Autodesk Fusion 360 part; units mm, degrees
note: some values were not read from the file. Set by a fixed rule: which sketch regions a step uses.
(part 12 of 20)
  spline S66 degree 5 poles (-5.1346, 28.5878) (-5.1347, 28.5879) (-5.1347, 28.5881) (-5.1348, 28.5884) (-5.1349, 28.5889) (-5.135, 28.5896) (-5.1352, 28.5905) (-5.1354, 28.5915) (-5.1356, 28.5925) (-5.1358, 28.5937) (-5.1361, 28.595) (-5.1363, 28.5964) (-5.1367, 28.5979) (-5.137, 28.5995) (-5.1374, 28.6012) (-5.1377, 28.603) (-5.1381, 28.6049) (-5.1386, 28.6069) (-5.139, 28.6089) (-5.1395, 28.6111) (-5.14, 28.6134) (-5.1406, 28.6158) (-5.1411, 28.6182) (-5.1417, 28.6208) (-5.1423, 28.6234) (-5.143, 28.6262) (-5.1436, 28.629) (-5.1443, 28.6319) (-5.145, 28.6349) (-5.1458, 28.6379) (-5.1465, 28.6411) (-5.1473, 28.6443) (-5.1481, 28.6477) (-5.149, 28.6511) (-5.1499, 28.6545) (-5.1508, 28.6581) (-5.1517, 28.6617) (-5.1527, 28.6655) (-5.1536, 28.6693) (-5.1546, 28.6731) (-5.1557, 28.6771) (-5.1567, 28.6811) (-5.1578, 28.6852) (-5.1589, 28.6893) (-5.1601, 28.6936) (-5.1613, 28.6979) (-5.1625, 28.7023) (-5.1637, 28.7067) (-5.1649, 28.7112) (-5.1662, 28.7158) (-5.1675, 28.7205) (-5.1689, 28.7252) (-5.1702, 28.73) (-5.1716, 28.7349) (-5.173, 28.7398) (-5.1745, 28.7448) (-5.176, 28.7498) (-5.1775, 28.7549) (-5.179, 28.7601) (-5.1806, 28.7654) (-5.1822, 28.7707) (-5.1838, 28.776) (-5.1854, 28.7815) (-5.1871, 28.7869) (-5.1888, 28.7925) (-5.1905, 28.7981) (-5.1923, 28.8038) (-5.1941, 28.8095) (-5.1959, 28.8153) (-5.1978, 28.8211) (-5.1996, 28.827) (-5.2015, 28.833) (-5.2035, 28.839) (-5.2054, 28.8451) (-5.2074, 28.8512) (-5.2094, 28.8573) (-5.2115, 28.8636) (-5.2136, 28.8699) (-5.2157, 28.8762) (-5.2178, 28.8826) (-5.22, 28.889) (-5.2222, 28.8955) (-5.2244, 28.9021) (-5.2266, 28.9087) (-5.2289, 28.9153) (-5.2312, 28.922) (-5.2336, 28.9288) (-5.2359, 28.9356) (-5.2383, 28.9424) (-5.2408, 28.9493) (-5.2432, 28.9563) (-5.2457, 28.9633) (-5.2482, 28.9703) (-5.2508, 28.9774) (-5.2533, 28.9846) (-5.2559, 28.9918) (-5.2586, 28.999) (-5.2612, 29.0063) (-5.2639, 29.0136) (-5.2666, 29.021) (-5.2694, 29.0284) (-5.2722, 29.0358) (-5.275, 29.0433) (-5.2778, 29.0509) (-5.2807, 29.0585) (-5.2836, 29.0661) (-5.2865, 29.0738) (-5.2895, 29.0815) (-5.2925, 29.0893) (-5.2955, 29.0971) (-5.2986, 29.105) (-5.3016, 29.1129) (-5.3047, 29.1208) (-5.3079, 29.1288) (-5.3111, 29.1368) (-5.3143, 29.1448) (-5.3175, 29.1529) (-5.3207, 29.1611) (-5.324, 29.1692) (-5.3273, 29.1775) (-5.3307, 29.1857) (-5.3341, 29.194) (-5.3375, 29.2023) (-5.3409, 29.2107) (-5.3444, 29.2191) (-5.3479, 29.2276) (-5.3514, 29.2361) (-5.355, 29.2446) (-5.3586, 29.2531) (-5.3622, 29.2617) (-5.3658, 29.2704) (-5.3695, 29.279) (-5.3732, 29.2878) (-5.377, 29.2965) (-5.3807, 29.3053) (-5.3846, 29.3141) (-5.3884, 29.3229) (-5.3922, 29.3318) (-5.3961, 29.3407) (-5.4001, 29.3497) (-5.404, 29.3587) (-5.408, 29.3677) (-5.412, 29.3767) (-5.4161, 29.3858) (-5.4201, 29.395) (-5.4242, 29.4041) (-5.4284, 29.4133) (-5.4325, 29.4225) (-5.4367, 29.4318) (-5.441, 29.441) (-5.4452, 29.4504) (-5.4495, 29.4597) (-5.4538, 29.4691) (-5.4582, 29.4785) (-5.4625, 29.4879) (-5.467, 29.4974) (-5.4714, 29.5069) (-5.4759, 29.5165) (-5.4804, 29.526) (-5.4849, 29.5356) (-5.4895, 29.5452) (-5.494, 29.5549) (-5.4987, 29.5646) (-5.5033, 29.5743) (-5.508, 29.584) (-5.5127, 29.5938) (-5.5175, 29.6036) (-5.5222, 29.6134) (-5.527, 29.6233) (-5.5319, 29.6332) (-5.5367, 29.6431) (-5.5416, 29.653) (-5.5466, 29.663) (-5.5515, 29.673) (-5.5565, 29.683) (-5.5615, 29.6931) (-5.5666, 29.7032) (-5.5717, 29.7133) (-5.5768, 29.7234) (-5.5819, 29.7336) (-5.5871, 29.7437) (-5.5923, 29.754) (-5.5975, 29.7642) (-5.6028, 29.7745) (-5.6081, 29.7847) (-5.6134, 29.7951) (-5.6188, 29.8054) (-5.6242, 29.8158) (-5.6296, 29.8262) (-5.635, 29.8366) (-5.6405, 29.847) (-5.646, 29.8575) (-5.6515, 29.868) (-5.6571, 29.8785) (-5.6627, 29.889) (-5.6683, 29.8996) (-5.674, 29.9102) (-5.6797, 29.9208) (-5.6854, 29.9314) (-5.6912, 29.9421) (-5.697, 29.9527) (-5.7028, 29.9634) (-5.7086, 29.9742) (-5.7145, 29.9849) (-5.7204, 29.9957) (-5.7263, 30.0065) (-5.7323, 30.0173) (-5.7383, 30.0281) (-5.7443, 30.039) (-5.7504, 30.0499) (-5.7565, 30.0608) (-5.7626, 30.0717) (-5.7688, 30.0826) (-5.7749, 30.0936) (-5.7811, 30.1046) (-5.7874, 30.1156) (-5.7937, 30.1266) (-5.8, 30.1377) (-5.8063, 30.1487) (-5.8127, 30.1598) (-5.8191, 30.1709) (-5.8255, 30.1821) (-5.8319, 30.1932) (-5.8384, 30.2044) (-5.8449, 30.2156) (-5.8515, 30.2268) (-5.8581, 30.238) (-5.8647, 30.2492) (-5.8713, 30.2605) (-5.878, 30.2718) (-5.8847, 30.2831) (-5.8914, 30.2944) (-5.8982, 30.3058) (-5.905, 30.3171) (-5.9118, 30.3285) (-5.9187, 30.3399) (-5.9255, 30.3513) (-5.9325, 30.3628) (-5.9394, 30.3742) (-5.9464, 30.3857) (-5.9534, 30.3972) (-5.959, 30.4064) (-5.9633, 30.4133) (-5.9661, 30.4179) (-5.9675, 30.4202) knots 0 0 0 0 0 0 0.00416667 0.00833333 0.0125 0.01666667 0.02083333 0.025 0.02916667 0.03333333 0.0375 0.04166667 0.04583333 0.05 0.05416667 0.05833333 0.0625 0.06666667 0.07083333 0.075 0.07916667 0.08333333 0.0875 0.09166667 0.09583333 0.1 0.10416667 0.10833333 0.1125 0.11666667 0.12083333 0.125 0.12916667 0.13333333 0.1375 0.14166667 0.14583333 0.15 0.15416667 0.15833333 0.1625 0.16666667 0.17083333 0.175 0.17916667 0.18333333 0.1875 0.19166667 0.19583333 0.2 0.20416667 0.20833333 0.2125 0.21666667 0.22083333 0.225 0.22916667 0.23333333 0.2375 0.24166667 0.24583333 0.25 0.25416667 0.25833333 0.2625 0.26666667 0.27083333 0.275 0.27916667 0.28333333 0.2875 0.29166667 0.29583333 0.3 0.30416667 0.30833333 0.3125 0.31666667 0.32083333 0.325 0.32916667 0.33333333 0.3375 0.34166667 0.34583333 0.35 0.35416667 0.35833333 0.3625 0.36666667 0.37083333 0.375 0.37916667 0.38333333 0.3875 0.39166667 0.39583333 0.4 0.40416667 0.40833333 0.4125 0.41666667 0.42083333 0.425 0.42916667 0.43333333 0.4375 0.44166667 0.44583333 0.45 0.45416667 0.45833333 0.4625 0.46666667 0.47083333 0.475 0.47916667 0.48333333 0.4875 0.49166667 0.49583333 0.5 0.50416667 0.50833333 0.5125 0.51666667 0.52083333 0.525 0.52916667 0.53333333 0.5375 0.54166667 0.54583333 0.55 0.55416667 0.55833333 0.5625 0.56666667 0.57083333 0.575 0.57916667 0.58333333 0.5875 0.59166667 0.59583333 0.6 0.60416667 0.60833333 0.6125 0.61666667 0.62083333 0.625 0.62916667 0.63333333 0.6375 0.64166667 0.64583333 0.65 0.65416667 0.65833333 0.6625 0.66666667 0.67083333 0.675 0.67916667 0.68333333 0.6875 0.69166667 0.69583333 0.7 0.70416667 0.70833333 0.7125 0.71666667 0.72083333 0.725 0.72916667 0.73333333 0.7375 0.74166667 0.74583333 0.75 0.75416667 0.75833333 0.7625 0.76666667 0.77083333 0.775 0.77916667 0.78333333 0.7875 0.79166667 0.79583333 0.8 0.80416667 0.80833333 0.8125 0.81666667 0.82083333 0.825 0.82916667 0.83333333 0.8375 0.84166667 0.84583333 0.85 0.85416667 0.85833333 0.8625 0.86666667 0.87083333 0.875 0.87916667 0.88333333 0.8875 0.89166667 0.89583333 0.9 0.90416667 0.90833333 0.9125 0.91666667 0.92083333 0.925 0.92916667 0.93333333 0.9375 0.94166667 0.94583333 0.95 0.95416667 0.95833333 0.9625 0.96666667 0.97083333 0.975 0.97916667 0.98333333 0.9875 0.99166667 0.99583333 1 1 1 1 1 1
  spline S67 degree 5 poles (-15.9204, 26.5997) (-15.9199, 26.597) (-15.9189, 26.5917) (-15.9174, 26.5837) (-15.9154, 26.5731) (-15.913, 26.5599) (-15.9105, 26.5467) (-15.908, 26.5335) (-15.9055, 26.5204) (-15.9029, 26.5073) (-15.9004, 26.4943) (-15.8979, 26.4812) (-15.8953, 26.4682) (-15.8927, 26.4553) (-15.8902, 26.4424) (-15.8876, 26.4295) (-15.885, 26.4166) (-15.8824, 26.4038) (-15.8798, 26.391) (-15.8771, 26.3783) (-15.8745, 26.3656) (-15.8719, 26.3529) (-15.8692, 26.3403) (-15.8666, 26.3276) (-15.8639, 26.3151) (-15.8612, 26.3025) (-15.8585, 26.29) (-15.8558, 26.2776) (-15.8531, 26.2651) (-15.8504, 26.2528) (-15.8477, 26.2404) (-15.8449, 26.2281) (-15.8422, 26.2158) (-15.8394, 26.2035) (-15.8367, 26.1913) (-15.8339, 26.1792) (-15.8311, 26.167) (-15.8283, 26.1549) (-15.8255, 26.1428) (-15.8227, 26.1308) (-15.8199, 26.1188) (-15.8171, 26.1069) (-15.8143, 26.095) (-15.8115, 26.0831) (-15.8086, 26.0712) (-15.8058, 26.0594) (-15.8029, 26.0477) (-15.8001, 26.0359) (-15.7972, 26.0242) (-15.7943, 26.0126) (-15.7914, 26.001) (-15.7886, 25.9894) (-15.7857, 25.9778) (-15.7828, 25.9663) (-15.7798, 25.9549) (-15.7769, 25.9435) (-15.774, 25.9321) (-15.7711, 25.9207) (-15.7682, 25.9094) (-15.7652, 25.8982) (-15.7623, 25.8869) (-15.7593, 25.8757) (-15.7564, 25.8646) (-15.7534, 25.8535) (-15.7504, 25.8424) (-15.7475, 25.8314) (-15.7445, 25.8204) (-15.7415, 25.8094) (-15.7385, 25.7985) (-15.7355, 25.7877) (-15.7325, 25.7768) (-15.7295, 25.766) (-15.7265, 25.7553) (-15.7235, 25.7446) (-15.7205, 25.7339) (-15.7175, 25.7233) (-15.7145, 25.7127) (-15.7114, 25.7022) (-15.7084, 25.6917) (-15.7054, 25.6812) (-15.7023, 25.6708) (-15.6993, 25.6604) (-15.6963, 25.6501) (-15.6932, 25.6398) (-15.6902, 25.6296) (-15.6871, 25.6194) (-15.6841, 25.6092) (-15.681, 25.5991) (-15.6779, 25.589) (-15.6749, 25.579) (-15.6718, 25.569) (-15.6688, 25.559) (-15.6657, 25.5491) (-15.6626, 25.5393) (-15.6596, 25.5294) (-15.6565, 25.5197) (-15.6534, 25.5099) (-15.6503, 25.5003) (-15.6473, 25.4906) (-15.6442, 25.481) (-15.6411, 25.4715) (-15.638, 25.462) (-15.635, 25.4525) (-15.6319, 25.4431) (-15.6288, 25.4337) (-15.6257, 25.4244) (-15.6227, 25.4151) (-15.6196, 25.4059) (-15.6165, 25.3967) (-15.6134, 25.3876) (-15.6104, 25.3785) (-15.6073, 25.3694) (-15.6042, 25.3604) (-15.6012, 25.3515) (-15.5981, 25.3426) (-15.595, 25.3337) (-15.592, 25.3249) (-15.5889, 25.3161) (-15.5859, 25.3074) (-15.5828, 25.2988) (-15.5798, 25.2901) (-15.5767, 25.2816) (-15.5737, 25.2731) (-15.5706, 25.2646) (-15.5676, 25.2562) (-15.5645, 25.2478) (-15.5615, 25.2394) (-15.5585, 25.2312) (-15.5555, 25.2229) (-15.5524, 25.2148) (-15.5494, 25.2066) (-15.5464, 25.1986) (-15.5434, 25.1905) (-15.5404, 25.1826) (-15.5374, 25.1746) (-15.5344, 25.1668) (-15.5315, 25.1589) (-15.5285, 25.1512) (-15.5255, 25.1434) (-15.5226, 25.1358) (-15.5196, 25.1282) (-15.5166, 25.1206) (-15.5137, 25.1131) (-15.5108, 25.1056) (-15.5078, 25.0982) (-15.5049, 25.0909) (-15.502, 25.0836) (-15.4991, 25.0763) (-15.4962, 25.0691) (-15.4933, 25.062) (-15.4905, 25.0549) (-15.4876, 25.0479) (-15.4848, 25.0409) (-15.4819, 25.034) (-15.4791, 25.0271) (-15.4762, 25.0203) (-15.4734, 25.0136) (-15.4706, 25.0069) (-15.4678, 25.0002) (-15.4651, 24.9936) (-15.4623, 24.9871) (-15.4595, 24.9806) (-15.4568, 24.9742) (-15.4541, 24.9679) (-15.4514, 24.9616) (-15.4486, 24.9553) (-15.446, 24.9492) (-15.4433, 24.943) (-15.4406, 24.937) (-15.438, 24.931) (-15.4353, 24.925) (-15.4327, 24.9192) (-15.4301, 24.9133) (-15.4275, 24.9076) (-15.425, 24.9019) (-15.4224, 24.8962) (-15.4199, 24.8907) (-15.4174, 24.8852) (-15.4149, 24.8797) (-15.4124, 24.8743) (-15.4099, 24.869) (-15.4075, 24.8637) (-15.405, 24.8585) (-15.4026, 24.8534) (-15.4002, 24.8483) (-15.3979, 24.8433) (-15.3955, 24.8384) (-15.3932, 24.8335) (-15.3909, 24.8287) (-15.3886, 24.8239) (-15.3863, 24.8193) (-15.3841, 24.8147) (-15.3819, 24.8101) (-15.3797, 24.8056) (-15.3775, 24.8012) (-15.3754, 24.7969) (-15.3733, 24.7926) (-15.3712, 24.7884) (-15.3691, 24.7843) (-15.3671, 24.7802) (-15.3651, 24.7763) (-15.3631, 24.7723) (-15.3611, 24.7685) (-15.3592, 24.7647) (-15.3573, 24.761) (-15.3554, 24.7574) (-15.3536, 24.7539) (-15.3518, 24.7504) (-15.35, 24.747) (-15.3482, 24.7437) (-15.3465, 24.7404) (-15.3449, 24.7372) (-15.3432, 24.7341) (-15.3416, 24.7311) (-15.34, 24.7282) (-15.3385, 24.7253) (-15.337, 24.7225) (-15.3355, 24.7198) (-15.3341, 24.7172) (-15.3327, 24.7147) (-15.3313, 24.7122) (-15.33, 24.7099) (-15.3287, 24.7076) (-15.3275, 24.7054) (-15.3263, 24.7033) (-15.3252, 24.7012) (-15.3241, 24.6993) (-15.323, 24.6974) (-15.322, 24.6956) (-15.321, 24.694) (-15.3201, 24.6924) (-15.3193, 24.6909) (-15.3184, 24.6895) (-15.3177, 24.6881) (-15.3169, 24.6869) (-15.3163, 24.6858) (-15.3157, 24.6848) (-15.3151, 24.6838) (-15.3146, 24.683) (-15.3142, 24.6822) (-15.3138, 24.6816) (-15.3135, 24.6812) (-15.3133, 24.6809) (-15.3132, 24.6807) (-15.3132, 24.6806) knots -1 -1 -1 -1 -1 -1 -0.99583333 -0.99166667 -0.9875 -0.98333333 -0.97916667 -0.975 -0.97083333 -0.96666667 -0.9625 -0.95833333 -0.95416667 -0.95 -0.94583333 -0.94166667 -0.9375 -0.93333333 -0.92916667 -0.925 -0.92083333 -0.91666667 -0.9125 -0.90833333 -0.90416667 -0.9 -0.89583333 -0.89166667 -0.8875 -0.88333333 -0.87916667 -0.875 -0.87083333 -0.86666667 -0.8625 -0.85833333 -0.85416667 -0.85 -0.84583333 -0.84166667 -0.8375 -0.83333333 -0.82916667 -0.825 -0.82083333 -0.81666667 -0.8125 -0.80833333 -0.80416667 -0.8 -0.79583333 -0.79166667 -0.7875 -0.78333333 -0.77916667 -0.775 -0.77083333 -0.76666667 -0.7625 -0.75833333 -0.75416667 -0.75 -0.74583333 -0.74166667 -0.7375 -0.73333333 -0.72916667 -0.725 -0.72083333 -0.71666667 -0.7125 -0.70833333 -0.70416667 -0.7 -0.69583333 -0.69166667 -0.6875 -0.68333333 -0.67916667 -0.675 -0.67083333 -0.66666667 -0.6625 -0.65833333 -0.65416667 -0.65 -0.64583333 -0.64166667 -0.6375 -0.63333333 -0.62916667 -0.625 -0.62083333 -0.61666667 -0.6125 -0.60833333 -0.60416667 -0.6 -0.59583333 -0.59166667 -0.5875 -0.58333333 -0.57916667 -0.575 -0.57083333 -0.56666667 -0.5625 -0.55833333 -0.55416667 -0.55 -0.54583333 -0.54166667 -0.5375 -0.53333333 -0.52916667 -0.525 -0.52083333 -0.51666667 -0.5125 -0.50833333 -0.50416667 -0.5 -0.49583333 -0.49166667 -0.4875 -0.48333333 -0.47916667 -0.475 -0.47083333 -0.46666667 -0.4625 -0.45833333 -0.45416667 -0.45 -0.44583333 -0.44166667 -0.4375 -0.43333333 -0.42916667 -0.425 -0.42083333 -0.41666667 -0.4125 -0.40833333 -0.40416667 -0.4 -0.39583333 -0.39166667 -0.3875 -0.38333333 -0.37916667 -0.375 -0.37083333 -0.36666667 -0.3625 -0.35833333 -0.35416667 -0.35 -0.34583333 -0.34166667 -0.3375 -0.33333333 -0.32916667 -0.325 -0.32083333 -0.31666667 -0.3125 -0.30833333 -0.30416667 -0.3 -0.29583333 -0.29166667 -0.2875 -0.28333333 -0.27916667 -0.275 -0.27083333 -0.26666667 -0.2625 -0.25833333 -0.25416667 -0.25 -0.24583333 -0.24166667 -0.2375 -0.23333333 -0.22916667 -0.225 -0.22083333 -0.21666667 -0.2125 -0.20833333 -0.20416667 -0.2 -0.19583333 -0.19166667 -0.1875 -0.18333333 -0.17916667 -0.175 -0.17083333 -0.16666667 -0.1625 -0.15833333 -0.15416667 -0.15 -0.14583333 -0.14166667 -0.1375 -0.13333333 -0.12916667 -0.125 -0.12083333 -0.11666667 -0.1125 -0.10833333 -0.10416667 -0.1 -0.09583333 -0.09166667 -0.0875 -0.08333333 -0.07916667 -0.075 -0.07083333 -0.06666667 -0.0625 -0.05833333 -0.05416667 -0.05 -0.04583333 -0.04166667 -0.0375 -0.03333333 -0.02916667 -0.025 -0.02083333 -0.01666667 -0.0125 -0.00833333 -0.00416667 0 0 0 0 0 0
  line L145 (-2.1183, -28.9679) -> (-2.1182, -28.9671)
  line L146 (-3.9507, -28.7745) -> (-3.9508, -28.7753)
  line L147 (25.6012, 13.7171) -> (25.6019, 13.7175)
  line L148 (26.1461, 12.6495) -> (26.1453, 12.6491)
  arc A66 (-5.0824, -28.2972) -> (-3.9106, -28.4828) centre (0, 0) ccw
  arc A67 (-3.7249, -30.7754) -> (-2.755, -30.8773) centre (0, 0) ccw
  spline S68 degree 5 poles (-16.3184, 24.0278) (-16.3185, 24.0279) (-16.3186, 24.0281) (-16.3188, 24.0283) (-16.3191, 24.0287) (-16.3195, 24.0294) (-16.32, 24.0301) (-16.3206, 24.0309) (-16.3212, 24.0317) (-16.3219, 24.0327) (-16.3227, 24.0338) (-16.3235, 24.035) (-16.3244, 24.0362) (-16.3253, 24.0375) (-16.3263, 24.0389) (-16.3274, 24.0404) (-16.3286, 24.042) (-16.3298, 24.0436) (-16.331, 24.0453) (-16.3324, 24.0471) (-16.3338, 24.049) (-16.3352, 24.051) (-16.3367, 24.053) (-16.3383, 24.0551) (-16.3399, 24.0572) (-16.3416, 24.0595) (-16.3434, 24.0618) (-16.3452, 24.0641) (-16.3471, 24.0666) (-16.349, 24.0691) (-16.351, 24.0717) (-16.353, 24.0743) (-16.3551, 24.077) (-16.3573, 24.0798) (-16.3595, 24.0826) (-16.3618, 24.0855) (-16.3641, 24.0884) (-16.3665, 24.0914) (-16.3689, 24.0945) (-16.3714, 24.0976) (-16.374, 24.1008) (-16.3766, 24.104) (-16.3792, 24.1073) (-16.3819, 24.1107) (-16.3847, 24.1141) (-16.3875, 24.1176) (-16.3904, 24.1211) (-16.3933, 24.1246) (-16.3963, 24.1283) (-16.3994, 24.1319) (-16.4024, 24.1356) (-16.4056, 24.1394) (-16.4088, 24.1432) (-16.412, 24.1471) (-16.4153, 24.151) (-16.4187, 24.155) (-16.4221, 24.159) (-16.4256, 24.1631) (-16.4291, 24.1672) (-16.4326, 24.1713) (-16.4362, 24.1755) (-16.4399, 24.1798) (-16.4436, 24.1841) (-16.4474, 24.1884) (-16.4512, 24.1928) (-16.455, 24.1972) (-16.459, 24.2017) (-16.4629, 24.2062) (-16.4669, 24.2107) (-16.471, 24.2153) (-16.4751, 24.2199) (-16.4793, 24.2246) (-16.4835, 24.2293) (-16.4877, 24.234) (-16.492, 24.2388) (-16.4964, 24.2436) (-16.5008, 24.2485) (-16.5053, 24.2534) (-16.5098, 24.2583) (-16.5143, 24.2633) (-16.5189, 24.2683) (-16.5236, 24.2733) (-16.5282, 24.2784) (-16.533, 24.2835) (-16.5378, 24.2887) (-16.5426, 24.2939) (-16.5475, 24.2991) (-16.5524, 24.3043) (-16.5574, 24.3096) (-16.5624, 24.3149) (-16.5675, 24.3203) (-16.5726, 24.3257) (-16.5778, 24.3311) (-16.583, 24.3365) (-16.5882, 24.342) (-16.5935, 24.3475) (-16.5989, 24.353) (-16.6043, 24.3586) (-16.6097, 24.3642) (-16.6152, 24.3698) (-16.6207, 24.3755) (-16.6263, 24.3812) (-16.6319, 24.3869) (-16.6376, 24.3926) (-16.6433, 24.3984) (-16.6491, 24.4042) (-16.6549, 24.41) (-16.6607, 24.4159) (-16.6666, 24.4218) (-16.6725, 24.4277) (-16.6785, 24.4336) (-16.6845, 24.4395) (-16.6906, 24.4455) (-16.6967, 24.4515) (-16.7029, 24.4576) (-16.7091, 24.4636) (-16.7153, 24.4697) (-16.7216, 24.4758) (-16.7279, 24.482) (-16.7343, 24.4881) (-16.7407, 24.4943) (-16.7472, 24.5005) (-16.7537, 24.5067) (-16.7602, 24.513) (-16.7668, 24.5192) (-16.7735, 24.5255) (-16.7801, 24.5319) (-16.7869, 24.5382) (-16.7936, 24.5446) (-16.8004, 24.5509) (-16.8073, 24.5573) (-16.8142, 24.5638) (-16.8211, 24.5702) (-16.8281, 24.5767) (-16.8351, 24.5831) (-16.8421, 24.5897) (-16.8492, 24.5962) (-16.8564, 24.6027) (-16.8636, 24.6093) (-16.8708, 24.6159) (-16.8781, 24.6225) (-16.8854, 24.6291) (-16.8927, 24.6357) (-16.9001, 24.6424) (-16.9075, 24.6491) (-16.915, 24.6558) (-16.9225, 24.6625) (-16.9301, 24.6692) (-16.9377, 24.6759) (-16.9453, 24.6827) (-16.953, 24.6895) (-16.9607, 24.6963) (-16.9685, 24.7031) (-16.9763, 24.7099) (-16.9841, 24.7168) (-16.992, 24.7236) (-16.9999, 24.7305) (-17.0079, 24.7374) (-17.0159, 24.7443) (-17.0239, 24.7512) (-17.032, 24.7582) (-17.0401, 24.7651) (-17.0483, 24.7721) (-17.0565, 24.7791) (-17.0647, 24.7861) (-17.073, 24.7931) (-17.0813, 24.8001) (-17.0897, 24.8071) (-17.0981, 24.8142) (-17.1065, 24.8212) (-17.115, 24.8283) (-17.1235, 24.8354) (-17.1321, 24.8425) (-17.1407, 24.8496) (-17.1493, 24.8568) (-17.158, 24.8639) (-17.1667, 24.8711) (-17.1754, 24.8782) (-17.1842, 24.8854) (-17.1931, 24.8926) (-17.2019, 24.8998) (-17.2108, 24.907) (-17.2198, 24.9142) (-17.2288, 24.9215) (-17.2378, 24.9287) (-17.2469, 24.936) (-17.2559, 24.9432) (-17.2651, 24.9505) (-17.2743, 24.9578) (-17.2835, 24.9651) (-17.2927, 24.9724) (-17.302, 24.9797) (-17.3113, 24.9871) (-17.3207, 24.9944) (-17.3301, 25.0017) (-17.3395, 25.0091) (-17.349, 25.0165) (-17.3585, 25.0238) (-17.3681, 25.0312) (-17.3777, 25.0386) (-17.3873, 25.046) (-17.397, 25.0534) (-17.4067, 25.0609) (-17.4164, 25.0683) (-17.4262, 25.0757) (-17.436, 25.0832) (-17.4458, 25.0906) (-17.4557, 25.0981) (-17.4657, 25.1055) (-17.4756, 25.113) (-17.4856, 25.1205) (-17.4956, 25.128) (-17.5057, 25.1355) (-17.5158, 25.143) (-17.526, 25.1505) (-17.5361, 25.158) (-17.5464, 25.1655) (-17.5566, 25.1731) (-17.5669, 25.1806) (-17.5772, 25.1881) (-17.5876, 25.1957) (-17.598, 25.2032) (-17.6084, 25.2108) (-17.6189, 25.2184) (-17.6294, 25.2259) (-17.6399, 25.2335) (-17.6505, 25.2411) (-17.6611, 25.2487) (-17.6718, 25.2563) (-17.6825, 25.2639) (-17.6932, 25.2715) (-17.7039, 25.2791) (-17.7147, 25.2867) (-17.7256, 25.2943) (-17.7364, 25.3019) (-17.7473, 25.3096) (-17.7583, 25.3172) (-17.7692, 25.3248) (-17.7802, 25.3325) (-17.7913, 25.3401) (-17.8023, 25.3477) (-17.8112, 25.3539) (-17.8179, 25.3584) (-17.8224, 25.3615) (-17.8246, 25.363) knots 0 0 0 0 0 0 0.00416667 0.00833333 0.0125 0.01666667 0.02083333 0.025 0.02916667 0.03333333 0.0375 0.04166667 0.04583333 0.05 0.05416667 0.05833333 0.0625 0.06666667 0.07083333 0.075 0.07916667 0.08333333 0.0875 0.09166667 0.09583333 0.1 0.10416667 0.10833333 0.1125 0.11666667 0.12083333 0.125 0.12916667 0.13333333 0.1375 0.14166667 0.14583333 0.15 0.15416667 0.15833333 0.1625 0.16666667 0.17083333 0.175 0.17916667 0.18333333 0.1875 0.19166667 0.19583333 0.2 0.20416667 0.20833333 0.2125 0.21666667 0.22083333 0.225 0.22916667 0.23333333 0.2375 0.24166667 0.24583333 0.25 0.25416667 0.25833333 0.2625 0.26666667 0.27083333 0.275 0.27916667 0.28333333 0.2875 0.29166667 0.29583333 0.3 0.30416667 0.30833333 0.3125 0.31666667 0.32083333 0.325 0.32916667 0.33333333 0.3375 0.34166667 0.34583333 0.35 0.35416667 0.35833333 0.3625 0.36666667 0.37083333 0.375 0.37916667 0.38333333 0.3875 0.39166667 0.39583333 0.4 0.40416667 0.40833333 0.4125 0.41666667 0.42083333 0.425 0.42916667 0.43333333 0.4375 0.44166667 0.44583333 0.45 0.45416667 0.45833333 0.4625 0.46666667 0.47083333 0.475 0.47916667 0.48333333 0.4875 0.49166667 0.49583333 0.5 0.50416667 0.50833333 0.5125 0.51666667 0.52083333 0.525 0.52916667 0.53333333 0.5375 0.54166667 0.54583333 0.55 0.55416667 0.55833333 0.5625 0.56666667 0.57083333 0.575 0.57916667 0.58333333 0.5875 0.59166667 0.59583333 0.6 0.60416667 0.60833333 0.6125 0.61666667 0.62083333 0.625 0.62916667 0.63333333 0.6375 0.64166667 0.64583333 0.65 0.65416667 0.65833333 0.6625 0.66666667 0.67083333 0.675 0.67916667 0.68333333 0.6875 0.69166667 0.69583333 0.7 0.70416667 0.70833333 0.7125 0.71666667 0.72083333 0.725 0.72916667 0.73333333 0.7375 0.74166667 0.74583333 0.75 0.75416667 0.75833333 0.7625 0.76666667 0.77083333 0.775 0.77916667 0.78333333 0.7875 0.79166667 0.79583333 0.8 0.80416667 0.80833333 0.8125 0.81666667 0.82083333 0.825 0.82916667 0.83333333 0.8375 0.84166667 0.84583333 0.85 0.85416667 0.85833333 0.8625 0.86666667 0.87083333 0.875 0.87916667 0.88333333 0.8875 0.89166667 0.89583333 0.9 0.90416667 0.90833333 0.9125 0.91666667 0.92083333 0.925 0.92916667 0.93333333 0.9375 0.94166667 0.94583333 0.95 0.95416667 0.95833333 0.9625 0.96666667 0.97083333 0.975 0.97916667 0.98333333 0.9875 0.99166667 0.99583333 1 1 1 1 1 1
  line L149 (26.1453, 12.6491) -> (25.8803, 12.5209)
  line L150 (-2.1182, -28.9671) -> (-2.0967, -28.6734)
  line L151 (25.3417, 13.578) -> (25.6012, 13.7171)
  arc A68 (29.6298, 9.1146) -> (29.3284, 10.0421) centre (0, 0) ccw
  line L152 (-0.9213, -29.0298) -> (-0.9213, -29.0307)
  arc A69 (-2.0967, -28.6734) -> (-0.9119, -28.7355) centre (0, 0) ccw
  line L153 (-3.9106, -28.4828) -> (-3.9507, -28.7745)
  arc A70 (27.0473, 9.7471) -> (26.6221, 10.8547) centre (0, 0) ccw
  arc A71 (-15.0758, 27.0873) -> (-15.9204, 26.5997) centre (0, 0) ccw
  arc A72 (-15.1575, 24.4297) -> (-16.1526, 23.7836) centre (0, 0) ccw
  line L154 (-0.9119, -28.7355) -> (-0.9213, -29.0298)
  arc A73 (28.5147, 12.1618) -> (28.1181, 13.0527) centre (0, 0) ccw
  spline S69 degree 5 poles (27.8945, 8.0948) (27.8946, 8.0948) (27.8948, 8.0948) (27.8951, 8.0949) (27.8956, 8.0951) (27.8963, 8.0953) (27.8971, 8.0956) (27.898, 8.0958) (27.8991, 8.0962) (27.9002, 8.0965) (27.9015, 8.0969) (27.9028, 8.0973) (27.9043, 8.0978) (27.9058, 8.0983) (27.9075, 8.0988) (27.9092, 8.0994) (27.9111, 8.1) (27.913, 8.1007) (27.915, 8.1013) (27.9172, 8.102) (27.9194, 8.1028) (27.9217, 8.1036) (27.9241, 8.1044) (27.9265, 8.1052) (27.9291, 8.1061) (27.9318, 8.107) (27.9345, 8.108) (27.9373, 8.109) (27.9402, 8.11) (27.9432, 8.1111) (27.9462, 8.1121) (27.9494, 8.1133) (27.9526, 8.1144) (27.9559, 8.1156) (27.9593, 8.1169) (27.9627, 8.1181) (27.9662, 8.1194) (27.9698, 8.1208) (27.9735, 8.1222) (27.9772, 8.1236) (27.9811, 8.125) (27.9849, 8.1265) (27.9889, 8.128) (27.9929, 8.1295) (27.997, 8.1311) (28.0012, 8.1327) (28.0054, 8.1344) (28.0097, 8.1361) (28.0141, 8.1378) (28.0185, 8.1395) (28.023, 8.1413) (28.0276, 8.1432) (28.0322, 8.145) (28.0369, 8.1469) (28.0416, 8.1488) (28.0464, 8.1508) (28.0513, 8.1528) (28.0562, 8.1548) (28.0612, 8.1569) (28.0663, 8.159) (28.0714, 8.1611) (28.0765, 8.1633) (28.0818, 8.1655) (28.087, 8.1677) (28.0924, 8.17) (28.0978, 8.1723) (28.1032, 8.1747) (28.1087, 8.177) (28.1143, 8.1795) (28.1199, 8.1819) (28.1256, 8.1844) (28.1313, 8.1869) (28.1371, 8.1895) (28.1429, 8.192) (28.1488, 8.1947) (28.1547, 8.1973) (28.1607, 8.2) (28.1667, 8.2027) (28.1728, 8.2055) (28.179, 8.2083) (28.1851, 8.2111) (28.1914, 8.214) (28.1977, 8.2169) (28.204, 8.2198) (28.2104, 8.2227) (28.2168, 8.2257) (28.2233, 8.2288) (28.2298, 8.2318) (28.2363, 8.2349) (28.2429, 8.2381) (28.2496, 8.2412) (28.2563, 8.2445) (28.263, 8.2477) (28.2698, 8.251) (28.2767, 8.2543) (28.2835, 8.2576) (28.2905, 8.261) (28.2974, 8.2644) (28.3044, 8.2678) (28.3115, 8.2713) (28.3186, 8.2748) (28.3257, 8.2784) (28.3329, 8.282) (28.3401, 8.2856) (28.3473, 8.2892) (28.3546, 8.2929) (28.3619, 8.2966) (28.3693, 8.3004) (28.3767, 8.3042) (28.3842, 8.308) (28.3917, 8.3118) (28.3992, 8.3157) (28.4068, 8.3196) (28.4144, 8.3236) (28.422, 8.3276) (28.4297, 8.3316) (28.4374, 8.3357) (28.4452, 8.3398) (28.4529, 8.3439) (28.4608, 8.348) (28.4686, 8.3522) (28.4765, 8.3565) (28.4845, 8.3607) (28.4924, 8.365) (28.5004, 8.3693) (28.5085, 8.3737) (28.5165, 8.3781) (28.5246, 8.3825) (28.5328, 8.387) (28.5409, 8.3915) (28.5491, 8.396) (28.5574, 8.4006) (28.5657, 8.4052) (28.574, 8.4098) (28.5823, 8.4145) (28.5907, 8.4192) (28.5991, 8.4239) (28.6075, 8.4287) (28.616, 8.4335) (28.6244, 8.4384) (28.633, 8.4432) (28.6415, 8.4481) (28.6501, 8.4531) (28.6587, 8.458) (28.6674, 8.463) (28.676, 8.4681) (28.6847, 8.4732) (28.6935, 8.4783) (28.7022, 8.4834) (28.711, 8.4886) (28.7199, 8.4938) (28.7287, 8.499) (28.7376, 8.5043) (28.7465, 8.5096) (28.7554, 8.515) (28.7644, 8.5203) (28.7734, 8.5257) (28.7824, 8.5312) (28.7914, 8.5367) (28.8005, 8.5422) (28.8096, 8.5477) (28.8187, 8.5533) (28.8279, 8.5589) (28.837, 8.5645) (28.8462, 8.5702) (28.8555, 8.5759) (28.8647, 8.5817) (28.874, 8.5874) (28.8833, 8.5932) (28.8926, 8.5991) (28.902, 8.605) (28.9113, 8.6109) (28.9207, 8.6168) (28.9302, 8.6228) (28.9396, 8.6288) (28.9491, 8.6348) (28.9586, 8.6409) (28.9681, 8.647) (28.9776, 8.6532) (28.9872, 8.6593) (28.9968, 8.6656) (29.0064, 8.6718) (29.016, 8.6781) (29.0257, 8.6844) (29.0354, 8.6907) (29.0451, 8.6971) (29.0548, 8.7035) (29.0646, 8.7099) (29.0743, 8.7164) (29.0841, 8.7229) (29.0939, 8.7295) (29.1037, 8.736) (29.1136, 8.7426) (29.1235, 8.7493) (29.1334, 8.7559) (29.1433, 8.7626) (29.1532, 8.7694) (29.1632, 8.7762) (29.1731, 8.783) (29.1831, 8.7898) (29.1932, 8.7967) (29.2032, 8.8036) (29.2132, 8.8105) (29.2233, 8.8175) (29.2334, 8.8245) (29.2435, 8.8315) (29.2537, 8.8386) (29.2638, 8.8457) (29.274, 8.8528) (29.2842, 8.86) (29.2944, 8.8671) (29.3046, 8.8744) (29.3148, 8.8816) (29.3251, 8.8889) (29.3354, 8.8963) (29.3457, 8.9036) (29.356, 8.911) (29.3663, 8.9184) (29.3766, 8.9259) (29.387, 8.9334) (29.3974, 8.9409) (29.4078, 8.9485) (29.4182, 8.956) (29.4286, 8.9637) (29.4391, 8.9713) (29.4495, 8.979) (29.46, 8.9867) (29.4705, 8.9945) (29.481, 9.0022) (29.4915, 9.0101) (29.5021, 9.0179) (29.5127, 9.0258) (29.5232, 9.0337) (29.5338, 9.0416) (29.5444, 9.0496) (29.555, 9.0576) (29.5657, 9.0657) (29.5763, 9.0737) (29.587, 9.0818) (29.5977, 9.09) (29.6084, 9.0981) (29.6169, 9.1047) (29.6234, 9.1096) (29.6276, 9.1129) (29.6298, 9.1146) knots 0 0 0 0 0 0 0.00416667 0.00833333 0.0125 0.01666667 0.02083333 0.025 0.02916667 0.03333333 0.0375 0.04166667 0.04583333 0.05 0.05416667 0.05833333 0.0625 0.06666667 0.07083333 0.075 0.07916667 0.08333333 0.0875 0.09166667 0.09583333 0.1 0.10416667 0.10833333 0.1125 0.11666667 0.12083333 0.125 0.12916667 0.13333333 0.1375 0.14166667 0.14583333 0.15 0.15416667 0.15833333 0.1625 0.16666667 0.17083333 0.175 0.17916667 0.18333333 0.1875 0.19166667 0.19583333 0.2 0.20416667 0.20833333 0.2125 0.21666667 0.22083333 0.225 0.22916667 0.23333333 0.2375 0.24166667 0.24583333 0.25 0.25416667 0.25833333 0.2625 0.26666667 0.27083333 0.275 0.27916667 0.28333333 0.2875 0.29166667 0.29583333 0.3 0.30416667 0.30833333 0.3125 0.31666667 0.32083333 0.325 0.32916667 0.33333333 0.3375 0.34166667 0.34583333 0.35 0.35416667 0.35833333 0.3625 0.36666667 0.37083333 0.375 0.37916667 0.38333333 0.3875 0.39166667 0.39583333 0.4 0.40416667 0.40833333 0.4125 0.41666667 0.42083333 0.425 0.42916667 0.43333333 0.4375 0.44166667 0.44583333 0.45 0.45416667 0.45833333 0.4625 0.46666667 0.47083333 0.475 0.47916667 0.48333333 0.4875 0.49166667 0.49583333 0.5 0.50416667 0.50833333 0.5125 0.51666667 0.52083333 0.525 0.52916667 0.53333333 0.5375 0.54166667 0.54583333 0.55 0.55416667 0.55833333 0.5625 0.56666667 0.57083333 0.575 0.57916667 0.58333333 0.5875 0.59166667 0.59583333 0.6 0.60416667 0.60833333 0.6125 0.61666667 0.62083333 0.625 0.62916667 0.63333333 0.6375 0.64166667 0.64583333 0.65 0.65416667 0.65833333 0.6625 0.66666667 0.67083333 0.675 0.67916667 0.68333333 0.6875 0.69166667 0.69583333 0.7 0.70416667 0.70833333 0.7125 0.71666667 0.72083333 0.725 0.72916667 0.73333333 0.7375 0.74166667 0.74583333 0.75 0.75416667 0.75833333 0.7625 0.76666667 0.77083333 0.775 0.77916667 0.78333333 0.7875 0.79166667 0.79583333 0.8 0.80416667 0.80833333 0.8125 0.81666667 0.82083333 0.825 0.82916667 0.83333333 0.8375 0.84166667 0.84583333 0.85 0.85416667 0.85833333 0.8625 0.86666667 0.87083333 0.875 0.87916667 0.88333333 0.8875 0.89166667 0.89583333 0.9 0.90416667 0.90833333 0.9125 0.91666667 0.92083333 0.925 0.92916667 0.93333333 0.9375 0.94166667 0.94583333 0.95 0.95416667 0.95833333 0.9625 0.96666667 0.97083333 0.975 0.97916667 0.98333333 0.9875 0.99166667 0.99583333 1 1 1 1 1 1
  arc A74 (25.8803, 12.5209) -> (25.3417, 13.578) centre (0, 0) ccw
  spline S70 degree 5 poles (-3.9508, -28.7753) (-3.9508, -28.7754) (-3.9508, -28.7756) (-3.9509, -28.7759) (-3.9509, -28.7764) (-3.951, -28.7772) (-3.9511, -28.778) (-3.9512, -28.779) (-3.9514, -28.7801) (-3.9515, -28.7813) (-3.9517, -28.7826) (-3.9518, -28.784) (-3.952, -28.7855) (-3.9522, -28.7871) (-3.9523, -28.7889) (-3.9525, -28.7907) (-3.9527, -28.7926) (-3.9529, -28.7946) (-3.9531, -28.7968) (-3.9534, -28.799) (-3.9536, -28.8013) (-3.9538, -28.8037) (-3.954, -28.8063) (-3.9543, -28.8089) (-3.9545, -28.8116) (-3.9547, -28.8144) (-3.955, -28.8172) (-3.9552, -28.8202) (-3.9555, -28.8233) (-3.9557, -28.8264) (-3.9559, -28.8297) (-3.9562, -28.833) (-3.9564, -28.8364) (-3.9567, -28.8399) (-3.9569, -28.8435) (-3.9572, -28.8472) (-3.9574, -28.8509) (-3.9577, -28.8547) (-3.9579, -28.8586) (-3.9581, -28.8626) (-3.9584, -28.8667) (-3.9586, -28.8709) (-3.9588, -28.8751) (-3.959, -28.8794) (-3.9593, -28.8838) (-3.9595, -28.8882) (-3.9597, -28.8928) (-3.9599, -28.8974) (-3.9601, -28.9021) (-3.9603, -28.9068) (-3.9605, -28.9117) (-3.9607, -28.9166) (-3.9609, -28.9215) (-3.961, -28.9266) (-3.9612, -28.9317) (-3.9614, -28.9369) (-3.9615, -28.9422) (-3.9617, -28.9475) (-3.9618, -28.9529) (-3.962, -28.9584) (-3.9621, -28.9639) (-3.9622, -28.9695) (-3.9623, -28.9752) (-3.9624, -28.9809) (-3.9625, -28.9867) (-3.9626, -28.9926) (-3.9627, -28.9985) (-3.9627, -29.0045) (-3.9628, -29.0106) (-3.9629, -29.0167) (-3.9629, -29.0229) (-3.9629, -29.0291) (-3.9629, -29.0355) (-3.963, -29.0418) (-3.963, -29.0483) (-3.9629, -29.0548) (-3.9629, -29.0613) (-3.9629, -29.068) (-3.9628, -29.0746) (-3.9628, -29.0814) (-3.9627, -29.0882) (-3.9626, -29.095) (-3.9626, -29.1019) (-3.9625, -29.1089) (-3.9623, -29.1159) (-3.9622, -29.123) (-3.9621, -29.1302) (-3.9619, -29.1374) (-3.9618, -29.1446) (-3.9616, -29.1519) (-3.9614, -29.1593) (-3.9612, -29.1667) (-3.961, -29.1742) (-3.9607, -29.1817) (-3.9605, -29.1893) (-3.9603, -29.197) (-3.96, -29.2047) (-3.9597, -29.2124) (-3.9594, -29.2202) (-3.9591, -29.2281) (-3.9588, -29.236) (-3.9584, -29.2439) (-3.9581, -29.2519) (-3.9577, -29.26) (-3.9573, -29.2681) (-3.9569, -29.2763) (-3.9565, -29.2845) (-3.9561, -29.2927) (-3.9556, -29.301) (-3.9552, -29.3094) (-3.9547, -29.3178) (-3.9542, -29.3263) (-3.9537, -29.3348) (-3.9532, -29.3433) (-3.9526, -29.3519) (-3.9521, -29.3606) (-3.9515, -29.3693) (-3.9509, -29.378) (-3.9503, -29.3868) (-3.9497, -29.3957) (-3.9491, -29.4045) (-3.9484, -29.4135) (-3.9478, -29.4225) (-3.9471, -29.4315) (-3.9464, -29.4406) (-3.9457, -29.4497) (-3.9449, -29.4588) (-3.9442, -29.468) (-3.9434, -29.4773) (-3.9426, -29.4866) (-3.9418, -29.4959) (-3.941, -29.5053) (-3.9402, -29.5147) (-3.9393, -29.5242) (-3.9384, -29.5337) (-3.9375, -29.5433) (-3.9366, -29.5529) (-3.9357, -29.5625) (-3.9348, -29.5722) (-3.9338, -29.5819) (-3.9328, -29.5917) (-3.9318, -29.6015) (-3.9308, -29.6113) (-3.9297, -29.6212) (-3.9287, -29.6312) (-3.9276, -29.6411) (-3.9265, -29.6512) (-3.9254, -29.6612) (-3.9243, -29.6713) (-3.9231, -29.6814) (-3.922, -29.6916) (-3.9208, -29.7018) (-3.9196, -29.7121) (-3.9183, -29.7224) (-3.9171, -29.7327) (-3.9158, -29.7431) (-3.9145, -29.7535) (-3.9132, -29.764) (-3.9119, -29.7744) (-3.9106, -29.785) (-3.9092, -29.7955) (-3.9078, -29.8061) (-3.9064, -29.8168) (-3.905, -29.8274) (-3.9035, -29.8382) (-3.9021, -29.8489) (-3.9006, -29.8597) (-3.8991, -29.8705) (-3.8976, -29.8814) (-3.896, -29.8923) (-3.8945, -29.9032) (-3.8929, -29.9142) (-3.8913, -29.9252) (-3.8896, -29.9362) (-3.888, -29.9473) (-3.8863, -29.9584) (-3.8846, -29.9696) (-3.8829, -29.9807) (-3.8812, -29.992) (-3.8795, -30.0032) (-3.8777, -30.0145) (-3.8759, -30.0258) (-3.8741, -30.0372) (-3.8722, -30.0486) (-3.8704, -30.06) (-3.8685, -30.0714) (-3.8666, -30.0829) (-3.8647, -30.0944) (-3.8628, -30.106) (-3.8608, -30.1176) (-3.8588, -30.1292) (-3.8568, -30.1409) (-3.8548, -30.1525) (-3.8527, -30.1643) (-3.8507, -30.176) (-3.8486, -30.1878) (-3.8464, -30.1996) (-3.8443, -30.2115) (-3.8422, -30.2233) (-3.84, -30.2353) (-3.8378, -30.2472) (-3.8356, -30.2592) (-3.8333, -30.2712) (-3.831, -30.2832) (-3.8288, -30.2953) (-3.8264, -30.3074) (-3.8241, -30.3195) (-3.8217, -30.3317) (-3.8194, -30.3439) (-3.817, -30.3561) (-3.8145, -30.3683) (-3.8121, -30.3806) (-3.8096, -30.3929) (-3.8071, -30.4053) (-3.8046, -30.4176) (-3.8021, -30.43) (-3.7995, -30.4424) (-3.797, -30.4549) (-3.7943, -30.4674) (-3.7917, -30.4799) (-3.7891, -30.4924) (-3.7864, -30.505) (-3.7837, -30.5176) (-3.781, -30.5302) (-3.7782, -30.5429) (-3.7755, -30.5556) (-3.7727, -30.5683) (-3.7699, -30.581) (-3.767, -30.5938) (-3.7642, -30.6066) (-3.7613, -30.6194) (-3.7584, -30.6323) (-3.7555, -30.6451) (-3.7525, -30.658) (-3.7496, -30.671) (-3.7466, -30.6839) (-3.7435, -30.6969) (-3.7405, -30.7099) (-3.7374, -30.723) (-3.7343, -30.736) (-3.7312, -30.7491) (-3.7287, -30.7596) (-3.7268, -30.7675) (-3.7256, -30.7728) (-3.7249, -30.7754) knots 0 0 0 0 0 0 0.00416667 0.00833333 0.0125 0.01666667 0.02083333 0.025 0.02916667 0.03333333 0.0375 0.04166667 0.04583333 0.05 0.05416667 0.05833333 0.0625 0.06666667 0.07083333 0.075 0.07916667 0.08333333 0.0875 0.09166667 0.09583333 0.1 0.10416667 0.10833333 0.1125 0.11666667 0.12083333 0.125 0.12916667 0.13333333 0.1375 0.14166667 0.14583333 0.15 0.15416667 0.15833333 0.1625 0.16666667 0.17083333 0.175 0.17916667 0.18333333 0.1875 0.19166667 0.19583333 0.2 0.20416667 0.20833333 0.2125 0.21666667 0.22083333 0.225 0.22916667 0.23333333 0.2375 0.24166667 0.24583333 0.25 0.25416667 0.25833333 0.2625 0.26666667 0.27083333 0.275 0.27916667 0.28333333 0.2875 0.29166667 0.29583333 0.3 0.30416667 0.30833333 0.3125 0.31666667 0.32083333 0.325 0.32916667 0.33333333 0.3375 0.34166667 0.34583333 0.35 0.35416667 0.35833333 0.3625 0.36666667 0.37083333 0.375 0.37916667 0.38333333 0.3875 0.39166667 0.39583333 0.4 0.40416667 0.40833333 0.4125 0.41666667 0.42083333 0.425 0.42916667 0.43333333 0.4375 0.44166667 0.44583333 0.45 0.45416667 0.45833333 0.4625 0.46666667 0.47083333 0.475 0.47916667 0.48333333 0.4875 0.49166667 0.49583333 0.5 0.50416667 0.50833333 0.5125 0.51666667 0.52083333 0.525 0.52916667 0.53333333 0.5375 0.54166667 0.54583333 0.55 0.55416667 0.55833333 0.5625 0.56666667 0.57083333 0.575 0.57916667 0.58333333 0.5875 0.59166667 0.59583333 0.6 0.60416667 0.60833333 0.6125 0.61666667 0.62083333 0.625 0.62916667 0.63333333 0.6375 0.64166667 0.64583333 0.65 0.65416667 0.65833333 0.6625 0.66666667 0.67083333 0.675 0.67916667 0.68333333 0.6875 0.69166667 0.69583333 0.7 0.70416667 0.70833333 0.7125 0.71666667 0.72083333 0.725 0.72916667 0.73333333 0.7375 0.74166667 0.74583333 0.75 0.75416667 0.75833333 0.7625 0.76666667 0.77083333 0.775 0.77916667 0.78333333 0.7875 0.79166667 0.79583333 0.8 0.80416667 0.80833333 0.8125 0.81666667 0.82083333 0.825 0.82916667 0.83333333 0.8375 0.84166667 0.84583333 0.85 0.85416667 0.85833333 0.8625 0.86666667 0.87083333 0.875 0.87916667 0.88333333 0.8875 0.89166667 0.89583333 0.9 0.90416667 0.90833333 0.9125 0.91666667 0.92083333 0.925 0.92916667 0.93333333 0.9375 0.94166667 0.94583333 0.95 0.95416667 0.95833333 0.9625 0.96666667 0.97083333 0.975 0.97916667 0.98333333 0.9875 0.99166667 0.99583333 1 1 1 1 1 1
  arc A75 (-0.4876, -30.9962) -> (0.4876, -30.9962) centre (0, 0) ccw
  line L155 (26.8948, 10.9659) -> (26.8955, 10.9662)
  spline S71 degree 5 poles (29.3284, 10.0421) (29.3257, 10.0422) (29.3203, 10.0423) (29.3122, 10.0425) (29.3014, 10.0428) (29.288, 10.0431) (29.2745, 10.0434) (29.2612, 10.0437) (29.2478, 10.044) (29.2345, 10.0442) (29.2212, 10.0445) (29.2079, 10.0447) (29.1947, 10.0449) (29.1815, 10.0451) (29.1683, 10.0453) (29.1551, 10.0454) (29.142, 10.0455) (29.129, 10.0457) (29.1159, 10.0458) (29.1029, 10.0458) (29.0899, 10.0459) (29.077, 10.046) (29.0641, 10.046) (29.0512, 10.046) (29.0383, 10.046) (29.0255, 10.046) (29.0127, 10.046) (29, 10.0459) (28.9872, 10.0458) (28.9745, 10.0458) (28.9619, 10.0457) (28.9493, 10.0456) (28.9367, 10.0454) (28.9241, 10.0453) (28.9116, 10.0451) (28.8991, 10.0449) (28.8867, 10.0448) (28.8743, 10.0445) (28.8619, 10.0443) (28.8495, 10.0441) (28.8372, 10.0438) (28.8249, 10.0436) (28.8127, 10.0433) (28.8005, 10.043) (28.7883, 10.0427) (28.7762, 10.0423) (28.7641, 10.042) (28.752, 10.0416) (28.74, 10.0412) (28.728, 10.0409) (28.716, 10.0405) (28.7041, 10.04) (28.6922, 10.0396) (28.6803, 10.0392) (28.6685, 10.0387) (28.6567, 10.0382) (28.645, 10.0377) (28.6333, 10.0372) (28.6216, 10.0367) (28.61, 10.0362) (28.5984, 10.0356) (28.5868, 10.0351) (28.5753, 10.0345) (28.5638, 10.0339) (28.5524, 10.0333) (28.541, 10.0327) (28.5296, 10.0321) (28.5183, 10.0314) (28.507, 10.0308) (28.4957, 10.0301) (28.4845, 10.0294) (28.4733, 10.0287) (28.4622, 10.028) (28.4511, 10.0273) (28.44, 10.0266) (28.429, 10.0258) (28.4181, 10.0251) (28.4071, 10.0243) (28.3962, 10.0235) (28.3854, 10.0227) (28.3745, 10.0219) (28.3638, 10.0211) (28.353, 10.0203) (28.3423, 10.0195) (28.3317, 10.0186) (28.321, 10.0177) (28.3105, 10.0169) (28.2999, 10.016) (28.2894, 10.0151) (28.279, 10.0142) (28.2686, 10.0133) (28.2582, 10.0123) (28.2479, 10.0114) (28.2376, 10.0104) (28.2274, 10.0095) (28.2172, 10.0085) (28.207, 10.0075) (28.1969, 10.0065) (28.1868, 10.0055) (28.1768, 10.0045) (28.1668, 10.0035) (28.1569, 10.0025) (28.147, 10.0014) (28.1372, 10.0004) (28.1274, 9.9993) (28.1176, 9.9983) (28.1079, 9.9972) (28.0982, 9.9961) (28.0886, 9.995) (28.079, 9.9939) (28.0695, 9.9928) (28.06, 9.9916) (28.0506, 9.9905) (28.0412, 9.9894) (28.0318, 9.9882) (28.0225, 9.9871) (28.0133, 9.9859) (28.004, 9.9847) (27.9949, 9.9836) (27.9858, 9.9824) (27.9767, 9.9812) (27.9677, 9.98) (27.9587, 9.9788) (27.9498, 9.9776) (27.9409, 9.9763) (27.9321, 9.9751) (27.9233, 9.9739) (27.9146, 9.9726) (27.9059, 9.9714) (27.8973, 9.9701) (27.8887, 9.9689) (27.8802, 9.9676) (27.8717, 9.9664) (27.8633, 9.9651) (27.8549, 9.9638) (27.8466, 9.9625) (27.8383, 9.9612) (27.8301, 9.9599) (27.8219, 9.9586) (27.8138, 9.9573) (27.8057, 9.956) (27.7977, 9.9547) (27.7898, 9.9534) (27.7819, 9.9521) (27.774, 9.9508) (27.7662, 9.9494) (27.7585, 9.9481) (27.7508, 9.9468) (27.7431, 9.9454) (27.7356, 9.9441) (27.728, 9.9428) (27.7206, 9.9414) (27.7132, 9.9401) (27.7058, 9.9387) (27.6985, 9.9374) (27.6912, 9.936) (27.6841, 9.9347) (27.6769, 9.9333) (27.6698, 9.932) (27.6628, 9.9306) (27.6559, 9.9293) (27.649, 9.9279) (27.6421, 9.9266) (27.6353, 9.9252) (27.6286, 9.9239) (27.622, 9.9225) (27.6154, 9.9212) (27.6088, 9.9199) (27.6023, 9.9185) (27.5959, 9.9172) (27.5896, 9.9158) (27.5833, 9.9145) (27.577, 9.9132) (27.5709, 9.9118) (27.5647, 9.9105) (27.5587, 9.9092) (27.5527, 9.9079) (27.5468, 9.9065) (27.5409, 9.9052) (27.5352, 9.9039) (27.5294, 9.9026) (27.5238, 9.9013) (27.5182, 9.9) (27.5127, 9.8987) (27.5072, 9.8974) (27.5018, 9.8962) (27.4965, 9.8949) (27.4912, 9.8936) (27.4861, 9.8924) (27.481, 9.8911) (27.4759, 9.8899) (27.4709, 9.8887) (27.466, 9.8874) (27.4612, 9.8862) (27.4564, 9.885) (27.4517, 9.8838) (27.4471, 9.8827) (27.4426, 9.8815) (27.4381, 9.8803) (27.4337, 9.8792) (27.4294, 9.878) (27.4252, 9.8769) (27.421, 9.8758) (27.4169, 9.8747) (27.4129, 9.8736) (27.409, 9.8725) (27.4051, 9.8715) (27.4013, 9.8704) (27.3976, 9.8694) (27.394, 9.8684) (27.3905, 9.8674) (27.387, 9.8664) (27.3837, 9.8654) (27.3804, 9.8645) (27.3772, 9.8635) (27.3741, 9.8626) (27.371, 9.8617) (27.3681, 9.8608) (27.3652, 9.86) (27.3625, 9.8591) (27.3598, 9.8583) (27.3572, 9.8575) (27.3547, 9.8568) (27.3523, 9.856) (27.3499, 9.8553) (27.3477, 9.8546) (27.3456, 9.8539) (27.3435, 9.8533) (27.3416, 9.8527) (27.3398, 9.8521) (27.338, 9.8515) (27.3364, 9.851) (27.3348, 9.8505) (27.3334, 9.85) (27.332, 9.8495) (27.3308, 9.8491) (27.3296, 9.8487) (27.3286, 9.8484) (27.3277, 9.8481) (27.3269, 9.8478) (27.3262, 9.8475) (27.3257, 9.8474) (27.3254, 9.8473) (27.3252, 9.8472) (27.3251, 9.8472) knots -1 -1 -1 -1 -1 -1 -0.99583333 -0.99166667 -0.9875 -0.98333333 -0.97916667 -0.975 -0.97083333 -0.96666667 -0.9625 -0.95833333 -0.95416667 -0.95 -0.94583333 -0.94166667 -0.9375 -0.93333333 -0.92916667 -0.925 -0.92083333 -0.91666667 -0.9125 -0.90833333 -0.90416667 -0.9 -0.89583333 -0.89166667 -0.8875 -0.88333333 -0.87916667 -0.875 -0.87083333 -0.86666667 -0.8625 -0.85833333 -0.85416667 -0.85 -0.84583333 -0.84166667 -0.8375 -0.83333333 -0.82916667 -0.825 -0.82083333 -0.81666667 -0.8125 -0.80833333 -0.80416667 -0.8 -0.79583333 -0.79166667 -0.7875 -0.78333333 -0.77916667 -0.775 -0.77083333 -0.76666667 -0.7625 -0.75833333 -0.75416667 -0.75 -0.74583333 -0.74166667 -0.7375 -0.73333333 -0.72916667 -0.725 -0.72083333 -0.71666667 -0.7125 -0.70833333 -0.70416667 -0.7 -0.69583333 -0.69166667 -0.6875 -0.68333333 -0.67916667 -0.675 -0.67083333 -0.66666667 -0.6625 -0.65833333 -0.65416667 -0.65 -0.64583333 -0.64166667 -0.6375 -0.63333333 -0.62916667 -0.625 -0.62083333 -0.61666667 -0.6125 -0.60833333 -0.60416667 -0.6 -0.59583333 -0.59166667 -0.5875 -0.58333333 -0.57916667 -0.575 -0.57083333 -0.56666667 -0.5625 -0.55833333 -0.55416667 -0.55 -0.54583333 -0.54166667 -0.5375 -0.53333333 -0.52916667 -0.525 -0.52083333 -0.51666667 -0.5125 -0.50833333 -0.50416667 -0.5 -0.49583333 -0.49166667 -0.4875 -0.48333333 -0.47916667 -0.475 -0.47083333 -0.46666667 -0.4625 -0.45833333 -0.45416667 -0.45 -0.44583333 -0.44166667 -0.4375 -0.43333333 -0.42916667 -0.425 -0.42083333 -0.41666667 -0.4125 -0.40833333 -0.40416667 -0.4 -0.39583333 -0.39166667 -0.3875 -0.38333333 -0.37916667 -0.375 -0.37083333 -0.36666667 -0.3625 -0.35833333 -0.35416667 -0.35 -0.34583333 -0.34166667 -0.3375 -0.33333333 -0.32916667 -0.325 -0.32083333 -0.31666667 -0.3125 -0.30833333 -0.30416667 -0.3 -0.29583333 -0.29166667 -0.2875 -0.28333333 -0.27916667 -0.275 -0.27083333 -0.26666667 -0.2625 -0.25833333 -0.25416667 -0.25 -0.24583333 -0.24166667 -0.2375 -0.23333333 -0.22916667 -0.225 -0.22083333 -0.21666667 -0.2125 -0.20833333 -0.20416667 -0.2 -0.19583333 -0.19166667 -0.1875 -0.18333333 -0.17916667 -0.175 -0.17083333 -0.16666667 -0.1625 -0.15833333 -0.15416667 -0.15 -0.14583333 -0.14166667 -0.1375 -0.13333333 -0.12916667 -0.125 -0.12083333 -0.11666667 -0.1125 -0.10833333 -0.10416667 -0.1 -0.09583333 -0.09166667 -0.0875 -0.08333333 -0.07916667 -0.075 -0.07083333 -0.06666667 -0.0625 -0.05833333 -0.05416667 -0.05 -0.04583333 -0.04166667 -0.0375 -0.03333333 -0.02916667 -0.025 -0.02083333 -0.01666667 -0.0125 -0.00833333 -0.00416667 0 0 0 0 0 0